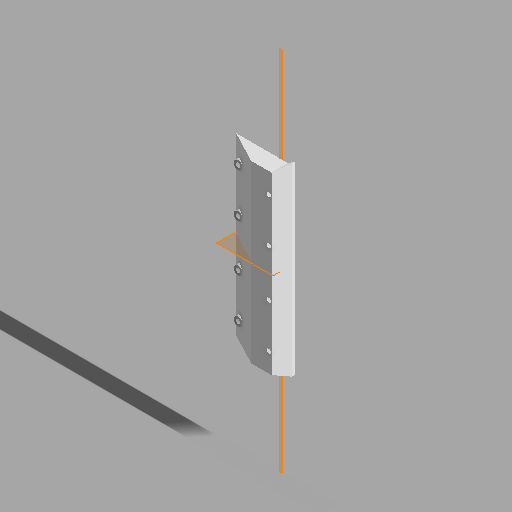
# Autodesk Inventor part: Порог_Левый
Saved by Autodesk Inventor 2025 (Build 290162000, 162)
## iProperties
Created: 2025-04-24
Part Number: Порог_Левый
Material: Типовые
Document SubType Name: Modeling
Designer: Artem Sannikov
Density: 1 g/cm^3
Appearance: По умолчанию
Author: Artem Sannikov
Autodesk Inventor part; units mm, degrees
ref_plane "YZ Plane" through (0, 0, 0) normal (1, 0, 0) x (0, 1, 0)
ref_plane "XZ Plane" through (0, 0, 0) normal (0, 1, 0) x (-1, 0, 0)
ref_plane "XY Plane" through (0, 0, 0) normal (0, 0, 1) x (1, 0, 0)
ref_plane "РабПлоскость1" through (0, 0, 0) normal (0, 0, 1) x (1, 0, 0)
sketch "Эскиз1" plane through (0, 0, 0) normal (0, 0, 1) x (1, 0, 0)
  line L0 (-41.5, 251.765) -> (-1.5, 251.765) construction
  line L1 (-41.5, 258.235) -> (-1.5, 258.235) construction
  line L2 (-41.5, 245) -> (-1.5, 245) construction
  line L3 (-41.5, 265) -> (-1.5, 265) construction
  line L4 (-21.5, 265) -> (-21.5, 245) construction
  line L5 (-55.5, 383.1594) -> (12.5, 383.1594)
  line L6 (12.5, 383.1594) -> (12.5, 126.8406)
  line L7 (12.5, 126.8406) -> (-55.5, 126.8406)
  line L8 (-55.5, 126.8406) -> (-55.5, 383.1594)
  line L9 (-55.5, 383.1594) -> (12.5, 126.8406) construction
  line L10 (12.5, 383.1594) -> (-55.5, 126.8406) construction
  point P0 (0, 0)
  point P1 (-21.5, 255)
  constraints: 14 end point, 5 midpoint, 2 parallel, 1 horizontal, 1 perpendicular, 1 other
extrude "Выдавливание1" add sketch "Эскиз1" along normal blind 4
sketch "Эскиз2" plane through (-55.5, 126.8406, 0) normal (0, -1, 0) x (1, 0, 0)
  line L0 (68, 0) -> (68, 24.2132) projected
  line L1 (0, 4) -> (68, 4) projected
  line L2 (38, 24.2132) -> (-8, 0) projected
  line L3 (68, 24.2132) -> (38, 24.2132) projected
  line L4 (68, 24.2132) -> (38, 24.2132) projected
  line L5 (68, 0) -> (68, 24.2132) projected
  line L6 (68, 0) -> (-8, 0) projected
  line L7 (38, 24.2132) -> (-8, 0) projected
  point P0 (55.5, 0)
extrude "Выдавливание2" add sketch "Эскиз2" against normal blind 1.5
sketch "Эскиз3" plane through (-55.5, 128.3406, 0) normal (-1, 0, 0) x (0, 0, 1)
  line L0 (0, 0) -> (4, 0) projected
  line L1 (4, 254.8188) -> (4, 0) projected
  line L2 (0, 254.8188) -> (4, 254.8188) projected
  line L3 (0, 254.8188) -> (0, 0) projected
  point P0 (0, -128.3406)
extrude "Выдавливание3" add sketch "Эскиз3" along normal up to surface (8 mm away)
ref_plane "РабПлоскость2" through (-55.5, 255.75, 0) normal (0, 1, 0) x (1, 0, 0)
mirror "Зеркальное отражение1" about plane through (-55.5, 255.75, 0) normal (0, 1, 0) of "Выдавливание2"
sketch "Эскиз4" plane through (-63.5, 128.3406, 4) normal (0, -1, 0) x (1, 0, 0)
  line L0 (0, -4) -> (7.5992, 0) projected
  line L1 (7.5992, 0) -> (0, 0) projected
  line L2 (0, 0) -> (0, -4) projected
  point P0 (63.5, -4)
extrude "Выдавливание4" cut sketch "Эскиз4" against normal through all
sketch "Эскиз5" plane through (12.5, 126.8406, 24.2132) normal (1, 0, 0) x (0, 0, -1)
  line L0 (24.2132, 0) -> (24.2132, 257.8188) projected
  line L1 (24.2132, 257.8188) -> (0, 257.8188) projected
  line L2 (0, 257.8188) -> (0, 256.3188) projected
  line L3 (0, 256.3188) -> (20.2132, 256.3188) projected
  line L4 (20.2132, 1.5) -> (20.2132, 256.3188) projected
  line L5 (0, 1.5) -> (20.2132, 1.5) projected
  line L6 (0, 0) -> (0, 1.5) projected
  line L7 (24.2132, 0) -> (0, 0) projected
  point P0 (24.2132, -126.8406)
ref_plane "РабПлоскость3" through (22.5, -10, -350) normal (1, 0, 0) x (0, 1, 0)
extrude "Выдавливание5" add sketch "Эскиз5" along normal up to surface (10 mm away)
sketch "Эскиз6" plane through (-55.9008, 383.1594, 4) normal (0, -1, 0) x (1, 0, 0)
  line L0 (38.4008, 53.3137) -> (58.2296, 53.3137) construction
  line L1 (68.4008, 53.3137) -> (58.2296, 53.3137) construction
  line L2 (68.4008, 53.3137) -> (68.4008, 0) construction
  line L3 (78.4008, 0) -> (0, 0) projected
  line L4 (38.4008, 53.3137) -> (38.4008, 0) construction
  line L5 (38.4008, 20.2132) -> (78.4008, 20.2132) projected
  line L6 (38.4008, 20.2132) -> (68.4008, 20.2132)
  line L7 (68.4008, 20.2132) -> (68.4008, 0)
  line L8 (68.4008, 0) -> (38.4008, 0)
  line L9 (38.4008, 0) -> (38.4008, 20.2132)
  point P0 (55.9008, -4)
  constraints: 12 end point, 2 parallel, 2 perpendicular, 2 point on line, 1 horizontal, 1 vertical
extrude "Выдавливание6" add sketch "Эскиз6" along normal up to surface (254.8188 mm away)
sketch "Эскиз7" plane through (-55.5, 128.3406, 0) normal (0, 1, 0) x (1, 0, 0)
  line L0 (38, -24.2132) -> (38, -4) projected
  line L1 (-0.4008, -4) -> (38, -4) projected
  line L2 (-0.4008, -4) -> (38, -24.2132) projected
  point P0 (55.5, 0)
extrude "Выдавливание7" add sketch "Эскиз7" along normal up to surface (254.8188 mm away)
sketch "Эскиз8" plane through (-55.5, 128.3406, 0) normal (0, 1, 0) x (1, 0, 0)
  point P0 (55.5, 0)
sketch "Эскиз9" plane through (-55.5, 128.3406, 0) normal (0, 1, 0) x (1, 0, 0)
  line L0 (68, -24.2132) -> (78, -4)
  line L1 (78, -4) -> (68, -4)
  line L2 (68, -4) -> (68, -24.2132)
  point P0 (55.5, 0)
  constraints: 6 end point, 1 perpendicular
extrude "Выдавливание8" add sketch "Эскиз9" along normal up to surface (254.8188 mm away)
sketch "Эскиз10" plane through (12.5, 383.1594, 24.2132) normal (0, -1, 0) x (1, 0, 0)
  line L0 (0, 0) -> (10, 0) projected
  line L1 (10, 0) -> (10, -20.2132) projected
  line L2 (10, -20.2132) -> (0, 0) projected
  point P0 (-12.5, -24.2132)
extrude "Выдавливание9" cut sketch "Эскиз10" along normal mid plane 776.5
sketch "Эскиз11" plane through (-63.5, 126.8406, 0) normal (0, -1, 0) x (1, 0, 0)
  line L0 (76, 0) -> (76, 24.2132) projected
  line L1 (86, 4) -> (76, 24.2132) projected
  line L2 (86, 0) -> (86, 4) projected
  line L3 (0, 0) -> (86, 0) projected
  point P0 (63.5, 0)
ref_plane "РабПлоскость4" through (22.5, 119.7696, -17) normal (0.5773502, 0.8164966, 0) x (0, 0, 1)
extrude "Выдавливание10" add sketch "Эскиз11" against normal up to surface surface through (22.5, 119.7696, -17) normal (0.5773502, 0.8164966, 0)
mirror "Зеркальное отражение2" about plane through (-55.5, 255.75, 0) normal (0, 1, 0) of "Выдавливание10"
sketch "Эскиз12" plane through (-17.5, 126.8406, 24.2132) normal (0, 0, 1) x (1, 0, 0)
  line L0 (36, -116.8406) -> (36, 373.1594) construction
  line L1 (26, -116.8406) -> (26, 373.1594) construction
  line L2 (-44, 393.1594) -> (-44, -136.8406) construction
  line L3 (-34, 393.1594) -> (-34, -136.8406) construction
  line L4 (36, 128.1594) -> (-44, 128.1594) construction
  circle A0 centre (26, 227.8188) radius 3.25
  circle A1 centre (26, 162.8188) radius 3.25
  line L5 (0, 257.8188) -> (30, 257.8188) projected
  circle A2 centre (-34, 162.8188) radius 3.25
  circle A3 centre (-34, 227.8188) radius 3.25
  circle A4 centre (26, 28.5) radius 3.25
  circle A5 centre (26, 93.5) radius 3.25
  circle A6 centre (-34, 93.5) radius 3.25
  circle A7 centre (-34, 28.5) radius 3.25
  point P0 (17.5, -126.8406)
  dimension "d23" = 10
  dimension "d24" = 10
  dimension "d25" = 6.5
  dimension "d26" = 6.5
  dimension "d27" = 65
  dimension "d28" = 30
  dimension "d29" = 6.5
  dimension "d30" = 6.5
  constraints: 8 centre point, 6 end point, 4 point on line, 4 symmetric about line, 2 midpoint, 2 parallel, 4 other
  measures "d23" distance between parallel lines of L0 L1
  measures "d24" distance between parallel lines of L2 L3
  measures "d25" diameter of A0
  measures "d26" diameter of A1
  measures "d27" distance of A1.centre A0.centre
  measures "d28" distance from line of L5 A0.centre
  measures "d29" diameter of A2
  measures "d30" diameter of A3
extrude "Выдавливание11" cut sketch "Эскиз12" along normal through all both and the other way through all
sketch "Эскиз13" plane through (0, 0, 0) normal (0, 0, -1) x (-1, 0, 0)
  circle A0 centre (51.5, 155.3406) radius 3.25 projected
  circle A1 centre (51.5, 155.3406) radius 6.5
  circle A2 centre (51.5, 220.3406) radius 3.25 projected
  circle A3 centre (51.5, 220.3406) radius 6.5
  circle A4 centre (51.5, 289.6594) radius 3.25 projected
  circle A5 centre (51.5, 289.6594) radius 6.5
  circle A6 centre (51.5, 354.6594) radius 3.25 projected
  circle A7 centre (51.5, 354.6594) radius 6.5
  point P0 (0, 0)
  dimension "d33" = 13
  dimension "d34" = 13
  dimension "d35" = 13
  dimension "d36" = 13
  constraints: 4 centre point, 4 coincident
  measures "d33" diameter of A1
  measures "d34" diameter of A3
  measures "d35" diameter of A5
  measures "d36" diameter of A7
extrude "Выдавливание12" add sketch "Эскиз13" against normal blind 9.25
